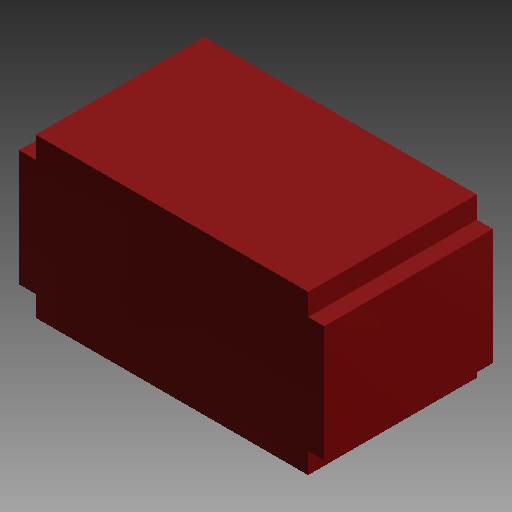
# Autodesk Inventor part: SK310A-TP
Saved by Autodesk Inventor 2018.2 (Build 222227000, 227)
## iProperties
Part Number: SK310A-TP
Material: Generic
Document SubType Name: Modeling
Designer: autocad
Appearance: SMA-SM, SK310A-TP
Author: autocad
Autodesk Inventor part; units mm, degrees
ref_plane "YZ Plane" through (0, 0, 0) normal (1, 0, 0) x (0, 1, 0)
ref_plane "XZ Plane" through (0, 0, 0) normal (0, 1, 0) x (-1, 0, 0)
ref_plane "XY Plane" through (0, 0, 0) normal (0, 0, 1) x (1, 0, 0)
sketch "SMA-SM, SK310A-TP_61" plane through (0, 0, 0) normal (0, 0, 1) x (1, 0, 0)
  line L0 (2.3876, 1.016) -> (2.667, 1.016)
  line L1 (2.667, 1.016) -> (2.667, -1.016)
  line L2 (2.667, -1.016) -> (2.3876, -1.016)
  line L3 (2.3876, -1.016) -> (2.3876, -1.377)
  line L4 (2.3876, -1.377) -> (-2.377, -1.377)
  line L5 (-2.377, -1.377) -> (-2.377, -1.016)
  line L6 (-2.377, -1.016) -> (-2.667, -1.016)
  line L7 (-2.667, -1.016) -> (-2.667, 1.016)
  line L8 (-2.667, 1.016) -> (-2.377, 1.016)
  line L9 (-2.377, 1.016) -> (-2.377, 1.397)
  line L10 (-2.377, 1.397) -> (2.3876, 1.397)
  line L11 (2.3876, 1.397) -> (2.3876, 1.016)
  constraints: 24 end point
extrude "Extrusion1" add sketch "SMA-SM, SK310A-TP_61" along normal blind 2.95
body "Solid1"
